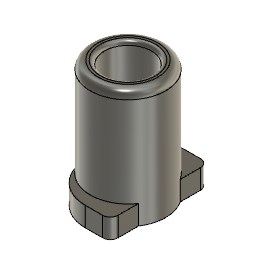
Messuhr_Einsatz_zylinderkopf_v1 (Autodesk Fusion 360 design; units mm, degrees)
part number: 2026-02-11-18-43-36-824
Autodesk Fusion 360 part; units mm, degrees
sketch "Skizze1" plane through (0, 0, 0) normal (0, 0, 1) x (1, 0, 0)
  circle A0 centre (0, 0) radius 6
  line L0 (-8, 12.5) -> (8, 12.5)
  line L1 (8, 12.5) -> (8, -12.5)
  line L2 (8, -12.5) -> (-8, -12.5)
  line L3 (-8, -12.5) -> (-8, 12.5)
  circle A1 centre (0, 0) radius 9.6
  line L4 (3.2696, -12.5) -> (3.2696, -5.0309) construction
  line L5 (3.2696, -5.0309) -> (8, -5.0309) construction
  line L6 (8, -5.0309) -> (8, -12.5) construction
  line L7 (8, -12.5) -> (3.2696, -12.5) construction
  line L8 (4, 5) -> (4, 12) construction
  line L9 (4, 12) -> (7, 12) construction
  line L10 (7, 12) -> (7, 5) construction
  line L11 (7, 5) -> (4, 5) construction
  line L12 (-6.9959, 3.6497) -> (-7.0141, 10.6497) construction
  line L13 (-7.0141, 10.6497) -> (-3.5098, 10.6588) construction
  line L14 (-3.5098, 10.6588) -> (-3.4917, 3.6588) construction
  line L15 (-3.4917, 3.6588) -> (-6.9959, 3.6497) construction
  dimension "d1" = 12
  dimension "d2" = 16
  dimension "d3" = 25
  dimension "d4" = 19.2
  dimension "d5" = 12.5
  dimension "d6" = 8
  dimension "d27" = 2
  dimension "d28" = 0
  dimension "d29" = 2
  dimension "d30" = 0
  dimension "d31" = 2
  dimension "d32" = 0
  text T0 "12" font "Arial" height 2 align centre middle in box 7.4691 x 4.7304 at (3.2696, -12.5) x (0, 1) y (1, 0) spacing 1
  text T1 "19,2" font "Arial" height 2 align centre middle in box 7 x 3 at (4, 5) x (0, 1) y (1, 0) spacing 1
  text T2 "30" font "Arial" height 2 align centre middle in box 7 x 3.5043 at (-6.9959, 3.6497) x (-0.00259, 0.999997) y (0.999997, 0.00259) spacing 1
  constraint coincident A0.centre A1.centre
  constraint horizontal L0
  constraint vertical L1
  constraint horizontal L2
  constraint vertical L3
  constraint coincident A0
  constraint coincident L1.end
  measures "d1" diameter of A0
  measures "d2" distance of L0.start L0.end
  measures "d3" distance of L0.start L2.end
  measures "d4" diameter of A1
  measures "d5" distance of L0 A0.centre
  measures "d6" distance of L3 A0.centre
extrude "Extrusion1" add sketch "Skizze1" along normal blind 30 contours L1 L3 A1
extrude "Extrusion2" add sketch "Skizze1" along normal blind 30 contours L1 A1
extrude "Extrusion3" add sketch "Skizze1" along normal blind 30 contours L3 A1
extrude "Extrusion4" add sketch "Skizze1" along normal blind 5 contours L0 L1 L3 A1
extrude "Extrusion5" add sketch "Skizze1" along normal blind 5 contours L1 L2 L3 A1
fillet "Abrundung1" radius 2 1 edges at (-8.9503, -3.4715, 30)
fillet "Abrundung2" radius 1 1 edges at (-5.594, 2.1697, 30)
fillet "Abrundung3" radius 1 1 edges at (-5.594, 2.1697, 0)
fillet "Abrundung4" radius 10 2 edges at (-8, 12.5, 2.5) (-8, -12.5, 2.5)
fillet "Abrundung5" radius 2 2 edges at (8, -12.5, 2.5) (8, 12.5, 2.5)
extrude "Extrusion6" cut sketch "Skizze1" along normal blind 2 text T0
extrude "Extrusion7" cut sketch "Skizze1" along normal blind 2.5 text T0
extrude "Extrusion8" cut sketch "Skizze1" along normal blind 2 text T1
extrude "Extrusion9" cut sketch "Skizze1" along normal blind 2 text T2
equation "d28 = '12'"
equation "d30 = '19,2'"
equation "d32 = '30'"
